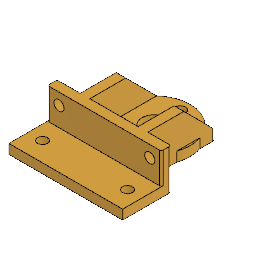
New2_Z_Nut_Bracket_1.0_F01 v7 (Autodesk Fusion 360 design; units mm, degrees)
Autodesk Fusion 360 part; units mm, degrees
sketch "スケッチ1" plane through (0, 0, 0) normal (0, 0, 1) x (1, 0, 0)
  line L0 (-17.5, 0) -> (-17.5, 34.6382)
  line L1 (-17.5, 34.6382) -> (17.5, 34.6382)
  line L2 (17.5, 34.6382) -> (17.5, 0)
  line L3 (-29.5, 0) -> (29.5, 0)
  line L4 (29.5, 0) -> (29.5, -25)
  line L5 (29.5, -25) -> (-29.5, -25)
  line L6 (-29.5, -25) -> (-29.5, 0)
  line L7 (-29.5, -5) -> (29.5, -5)
  line L8 (-12.5, 0) -> (-12.5, 34.6382)
  line L9 (12.5, 0) -> (12.5, 34.6382)
  circle A0 centre (22, -15) radius 2.6
  circle A1 centre (-22, -15) radius 2.6
  line L10 (29.5, -12.4) -> (22, -12.4)
  line L11 (29.5, -17.6) -> (22, -17.6)
  line L12 (-29.5, -12.4) -> (-22, -12.4)
  line L13 (-29.5, -17.6) -> (-22, -17.6)
  line L14 (0, 34.6382) -> (0, 0) construction
  circle A2 centre (0, 21) radius 18.5
  line L15 (-18.5, 21) -> (18.5, 21) construction
  circle A3 centre (0, 21) radius 6.5
  circle A4 centre (0, 7.7) radius 2.75
  circle A5 centre (0, 34.3) radius 2.75
  point P0 (0, 21)
  point P1 (0, 7.7)
  point P2 (0, 7.7)
  point P3 (0, 7.7)
  point P4 (0, 34.3)
  dimension "d2" = 25
  dimension "d3" = 5
  dimension "d4" = 35
  dimension "d5" = 59
  dimension "d6" = 17.5
  dimension "d7" = 5
  dimension "d8" = 5
  dimension "d9" = 5.2
  dimension "d10" = 5.2
  dimension "d11" = 7.5
  dimension "d12" = 7.5
  dimension "d13" = 10
  dimension "d14" = 10
  dimension "d67" = 21
  dimension "d72" = 37
  dimension "d90" = 13
  dimension "d91" = 5.5
  dimension "d93" = 5.5
  dimension "d97" = 13.3
  dimension "d98" = 13.3
  constraint vertical L0
  constraint perpendicular L0 L1
  constraint perpendicular L1 L2
  constraint perpendicular L2 L3
  constraint perpendicular L3 L4
  constraint perpendicular L4 L5
  constraint perpendicular L5 L6
  constraint coincident L6 L7.start
  constraint coincident L4 L7.end
  constraint perpendicular L4 L7
  constraint midpoint L14.end L3
  constraint coincident L2.end L3
  constraint coincident L3 L8.start
  constraint coincident L1 L8.end
  constraint perpendicular L1 L8
  constraint coincident L3 L9.start
  constraint coincident L1 L9.end
  constraint perpendicular L1 L9
  constraint coincident L4 L10.start
  constraint coincident A0 L10.end
  constraint perpendicular L4 L10
  constraint coincident L4 L11.start
  constraint coincident A0 L11.end
  constraint perpendicular L4 L11
  constraint coincident L6 L12.start
  constraint coincident A1 L12.end
  constraint perpendicular L6 L12
  constraint coincident L6 L13.start
  constraint coincident A1 L13.end
  constraint perpendicular L6 L13
  constraint tangent A1 L12
  constraint tangent A1 L13
  constraint tangent A0 L10
  constraint tangent A0 L11
  constraint midpoint L1 L14.start
  constraint coincident L14.end origin
  constraint coincident L14 P0
  constraint coincident P0 A2.centre
  constraint coincident L14 P3
  constraint coincident P3 P2
  constraint coincident A2 L15.start
  constraint coincident A2 L15.end
  constraint perpendicular L2 L15
  constraint coincident P0 L15
  constraint coincident L14 P4
  constraint concentric A2 A3
  constraint coincident P4 A5.centre
  constraint coincident L8.end A2
  measures "d2" vertical distance of L3.end L4.end
  measures "d3" distance of L3 L7
  measures "d4" distance of L0 L2
  measures "d5" horizontal distance of L4.end L5.end
  measures "d6" distance of L14.end L0
  measures "d7" distance of L0 L8
  measures "d8" distance of L2 L9
  measures "d9" diameter of A0
  measures "d10" diameter of A1
  measures "d11" distance of L4 A0.centre
  measures "d12" distance of L6 A1.centre
  measures "d13" distance of L5 A0.centre
  measures "d14" distance of L5 A1.centre
  measures "d67" distance of L3 P0
  measures "d72" diameter of A2
  measures "d90" diameter of A3
  measures "d91" diameter of A4
  measures "d93" diameter of A5
  measures "d97" distance of P3 P0
  measures "d98" distance of P4 P0
extrude "押し出し1" add sketch "スケッチ1" along normal blind 5 contours L3 L4 L6 L7 | L0 L3 L8 A2 | L0 A2 | L0 L8 A2 | L3 L8 L9 A2 | L0 L1 A2 | L1 L8 L9 A2 A5 | L4 L5 L6 L7 A0 A1 L10 L11 L12 L13 | L2 L3 L9 A2 | L1 A2 A5 | L2 L9 A2 | L6 A1 L12 L13 | L1 L2 A2 | L2 A2 | L4 A0 L10 L11
extrude "押し出し2" add sketch "スケッチ1" along normal blind 21 contours L3 L4 L6 L7
extrude "押し出し3" add sketch "スケッチ1" along normal up to surface (21 mm away) contours L0 L3 L8 A2 | L0 L8 A2 | L0 L1 A2 | L2 L3 L9 A2 | L2 L9 A2 | L1 L2 A2
hole "穴1" at (23.5, -5, 15) direction (0, 1, 0) diameter 5.2 depth 6 tip angle 118
hole "穴2" at (-23.5, -5, 15) direction (0, 1, 0) diameter 5.2 depth 6 tip angle 118
fillet "フィレット1" radius 1 6 edges at (29.5, -5, 13) (29.5, 0, 10.5) (17.5, 34.6382, 10.5) (-17.5, 34.6382, 10.5) (-29.5, 0, 10.5) (-29.5, -5, 13)
sketch "Sketch3" plane through (12.5, 0, 0) normal (-1, 0, 0) x (0, -1, 0)
  line L0 (-34.6382, 5) -> (0, 5)
  line L1 (0, 5) -> (0, 21)
  line L2 (0, 21) -> (-34.6382, 21)
  line L3 (-34.6382, 21) -> (-34.6382, 5)
  line L4 (-34.6382, 5) -> (-18.6382, 21)
  dimension "d99" = 45
  constraint coincident L0.start L3.end
  constraint coincident L2 L4.end
  measures "d99" angle of L2 L4
extrude "Extrude6" cut sketch "Sketch3" along normal through all and the other way through all contours L2 L3 L4
equation "d6 = d4 / 2"
